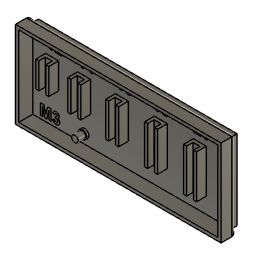
M3 Reference Caliper From 12 v2 (Autodesk Fusion 360 design; units mm, degrees)
Autodesk Fusion 360 part; units mm, degrees
note: some values were not read from the file. Chosen so that the rebuilt part matches the saved one: which bodies a step acts on; which pieces of a blend or face edit are solid.
sketch "Schizzo1" plane through (0, 0, 0) normal (0, 1, 0) x (1, 0, 0)
  line L0 (-43.0702, -47.1256) -> (51.9298, -47.1256)
  line L1 (51.9298, -47.1256) -> (51.9298, -7.1256)
  line L2 (51.9298, -7.1256) -> (-43.0702, -7.1256)
  line L3 (-43.0702, -7.1256) -> (-43.0702, -47.1256)
  line L4 (-34.9398, -37.9923) -> (-30.6504, -37.9923) construction
  line L5 (-30.6504, -37.9923) -> (-30.6504, -43.6096) construction
  line L6 (-30.6504, -43.6096) -> (-34.9398, -43.6096) construction
  line L7 (-34.9398, -43.6096) -> (-34.9398, -37.9923) construction
  line L8 (-20.4362, -37.9923) -> (-16.447, -37.9923) construction
  line L9 (-16.447, -37.9923) -> (-16.447, -43.6096) construction
  line L10 (-16.447, -43.6096) -> (-20.4362, -43.6096) construction
  line L11 (-20.4362, -43.6096) -> (-20.4362, -37.9923) construction
  line L12 (-2.7087, -37.9923) -> (2.1333, -37.9923) construction
  line L13 (2.1333, -37.9923) -> (2.1333, -43.6096) construction
  line L14 (2.1333, -43.6096) -> (-2.7087, -43.6096) construction
  line L15 (-2.7087, -43.6096) -> (-2.7087, -37.9923) construction
  line L16 (14.1885, -37.9923) -> (20.8281, -37.9923) construction
  line L17 (20.8281, -37.9923) -> (20.8281, -43.6096) construction
  line L18 (20.8281, -43.6096) -> (14.1885, -43.6096) construction
  line L19 (14.1885, -43.6096) -> (14.1885, -37.9923) construction
  line L20 (32.7115, -37.9923) -> (40.1532, -37.9923) construction
  line L21 (40.1532, -37.9923) -> (40.1532, -43.6096) construction
  line L22 (40.1532, -43.6096) -> (32.7115, -43.6096) construction
  line L23 (32.7115, -43.6096) -> (32.7115, -37.9923) construction
  line L24 (-35.6629, -35.9305) -> (-29.6629, -35.9305)
  line L25 (-29.6629, -35.9305) -> (-29.6629, -23.9305)
  line L26 (-29.6629, -23.9305) -> (-35.6629, -23.9305)
  line L27 (-35.6629, -23.9305) -> (-35.6629, -35.9305)
  line L28 (-32.6629, -35.9305) -> (-32.6629, -23.9305) construction
  line L29 (-31.0629, -23.9305) -> (-34.2629, -23.9305)
  line L30 (-34.2629, -23.9305) -> (-34.2629, -35.9305)
  line L31 (-34.2629, -35.9305) -> (-31.0629, -35.9305)
  line L32 (-31.0629, -35.9305) -> (-31.0629, -23.9305)
  line L33 (-31.0629, -23.9305) -> (-34.2629, -35.9305) construction
  line L34 (-34.2629, -23.9305) -> (-31.0629, -35.9305) construction
  line L35 (-14.8624, -21.9305) -> (-20.8624, -21.9305)
  line L36 (-19.4624, -21.9305) -> (-16.2624, -35.9305) construction
  line L37 (-16.2624, -21.9305) -> (-19.4624, -21.9305)
  line L38 (-16.2624, -35.9305) -> (-16.2624, -21.9305)
  line L39 (-19.4624, -21.9305) -> (-19.4624, -35.9305)
  line L40 (-16.2624, -21.9305) -> (-19.4624, -35.9305) construction
  line L41 (-17.8624, -35.9305) -> (-17.8624, -21.9305) construction
  line L42 (-20.8624, -35.9305) -> (-14.8624, -35.9305)
  line L43 (-20.8624, -21.9305) -> (-20.8624, -35.9305)
  line L44 (-14.8624, -35.9305) -> (-14.8624, -21.9305)
  line L45 (-19.4624, -35.9305) -> (-16.2624, -35.9305)
  line L46 (1.2, -35.9305) -> (1.2, -19.9305)
  line L47 (-3.4, -19.9305) -> (-3.4, -35.9305)
  line L48 (2.6, -35.9305) -> (2.6, -19.9305)
  line L49 (-3.4, -35.9305) -> (2.6, -35.9305)
  line L50 (1.2, -19.9305) -> (-2, -35.9305) construction
  line L51 (1.2, -19.9305) -> (-2, -19.9305)
  line L52 (-2, -19.9305) -> (-2, -35.9305)
  line L53 (-2, -19.9305) -> (1.2, -35.9305) construction
  line L54 (2.6, -19.9305) -> (-3.4, -19.9305)
  line L55 (-0.4, -35.9305) -> (-0.4, -19.9305) construction
  line L56 (-2, -35.9305) -> (1.2, -35.9305)
  line L57 (16.0001, -35.9305) -> (19.2001, -35.9305)
  line L58 (16.0001, -17.9305) -> (16.0001, -35.9305)
  line L59 (14.6001, -35.9305) -> (20.6001, -35.9305)
  line L60 (19.2001, -35.9305) -> (19.2001, -17.9305)
  line L61 (19.2001, -17.9305) -> (16.0001, -35.9305) construction
  line L62 (20.6001, -17.9305) -> (14.6001, -17.9305)
  line L63 (17.6001, -35.9305) -> (17.6001, -17.9305) construction
  line L64 (14.6001, -17.9305) -> (14.6001, -35.9305)
  line L65 (19.2001, -17.9305) -> (16.0001, -17.9305)
  line L66 (16.0001, -17.9305) -> (19.2001, -35.9305) construction
  line L67 (20.6001, -35.9305) -> (20.6001, -17.9305)
  line L68 (-43.0702, -35.9305) -> (51.9298, -35.9305) construction
  line L69 (32.6049, -35.9305) -> (38.6049, -35.9305)
  line L70 (37.2049, -15.9305) -> (34.0049, -35.9305) construction
  line L71 (38.6049, -35.9305) -> (38.6049, -15.9305)
  line L72 (32.6049, -15.9305) -> (32.6049, -35.9305)
  line L73 (37.2049, -35.9305) -> (37.2049, -15.9305)
  line L74 (37.2049, -15.9305) -> (34.0049, -15.9305)
  line L75 (35.6049, -35.9305) -> (35.6049, -15.9305) construction
  line L76 (34.0049, -15.9305) -> (34.0049, -35.9305)
  line L77 (34.0049, -35.9305) -> (37.2049, -35.9305)
  line L78 (34.0049, -15.9305) -> (37.2049, -35.9305) construction
  line L79 (38.6049, -15.9305) -> (32.6049, -15.9305)
  line L80 (-43.0702, -43.6096) -> (51.9298, -43.6096) construction
  line L81 (50.4298, -45.6256) -> (50.4298, -8.6256)
  line L82 (50.4298, -8.6256) -> (-41.5702, -8.6256)
  line L83 (-41.5702, -8.6256) -> (-41.5702, -45.6256)
  line L84 (-41.5702, -45.6256) -> (50.4298, -45.6256)
  line L85 (-38, -10) -> (-25, -10) construction
  line L86 (-25, -10) -> (-25, -15) construction
  line L87 (-25, -15) -> (-38, -15) construction
  line L88 (-38, -15) -> (-38, -10) construction
  line L89 (-43.0702, -37.9923) -> (50.4298, -37.9923) construction
  circle A0 centre (-17.6072, -12.9667) radius 1.5
  circle A1 centre (-17.6072, -12.9667) radius 2
  point P0 (-32.6629, -29.9305)
  point P1 (-17.8624, -28.9305)
  point P2 (-0.4, -27.9305)
  point P3 (17.6001, -26.9305)
  point P4 (35.6049, -25.9305)
  dimension "d1" = 40
  dimension "d2" = 5
  dimension "d3" = 5
  dimension "d4" = 5
  dimension "d5" = 5
  dimension "d6" = 5
  dimension "d7" = 6
  dimension "d8" = 12
  dimension "d9" = 3.2
  dimension "d21" = 6
  dimension "d22" = 14
  dimension "d23" = 3.2
  dimension "d24" = 6
  dimension "d25" = 16
  dimension "d26" = 3.2
  dimension "d27" = 6
  dimension "d28" = 18
  dimension "d29" = 3.2
  dimension "d30" = 6
  dimension "d31" = 20
  dimension "d32" = 3.2
  dimension "d33" = 95
  dimension "d34" = -1.5
  dimension "d37" = 5
  dimension "d40" = 3
  dimension "d41" = 4
  text T0 "12" font "Arial" height 5 bold align left top in box 4.2894 x 5.6173 at (-34.9398, -37.9923) x (1, 0) y (0, -1) spacing 1
  text T1 "14" font "Arial" height 5 bold align left top in box 3.9891 x 5.6173 at (-20.4362, -37.9923) x (1, 0) y (0, -1) spacing 1
  text T2 "16" font "Arial" height 5 bold align left top in box 4.842 x 5.6173 at (-2.7087, -37.9923) x (1, 0) y (0, -1) spacing 1
  text T3 "18" font "Arial" height 5 bold align left top in box 6.6397 x 5.6173 at (14.1885, -37.9923) x (1, 0) y (0, -1) spacing 1
  text T4 "20" font "Arial" height 5 bold align left top in box 7.4417 x 5.6173 at (32.7115, -37.9923) x (1, 0) y (0, -1) spacing 1
  text T5 "M3" font "Arial" height 5 bold align left top in box 13 x 5 at (-38, -10) x (1, 0) y (0, -1) spacing 1
  constraint horizontal L0
  constraint vertical L1
  constraint horizontal L2
  constraint vertical L3
  constraint horizontal L24
  constraint vertical L25
  constraint horizontal L26
  constraint vertical L27
  constraint midpoint L24 L28.start
  constraint midpoint L26 L28.end
  constraint horizontal L29
  constraint perpendicular L29 L30
  constraint parallel L29 L31
  constraint parallel L30 L32
  constraint coincident L33 P0
  constraint coincident L34 P0
  constraint coincident L26 L29.start
  constraint midpoint L28 P0
  constraint horizontal L42
  constraint vertical L44
  constraint horizontal L35
  constraint vertical L43
  constraint midpoint L41.start L42
  constraint midpoint L41.end L35
  constraint horizontal L37
  constraint perpendicular L37 L39
  constraint parallel L37 L45
  constraint parallel L38 L39
  constraint coincident P1 L40
  constraint coincident P1 L36
  constraint coincident L37.start L35
  constraint midpoint P1 L41
  constraint horizontal L49
  constraint vertical L48
  constraint horizontal L54
  constraint vertical L47
  constraint midpoint L55.start L49
  constraint midpoint L55.end L54
  constraint horizontal L51
  constraint perpendicular L51 L52
  constraint parallel L51 L56
  constraint parallel L46 L52
  constraint coincident P2 L50
  constraint coincident P2 L53
  constraint coincident L46.end L54
  constraint midpoint P2 L55
  constraint horizontal L59
  constraint vertical L67
  constraint horizontal L62
  constraint vertical L64
  constraint midpoint L63.start L59
  constraint midpoint L63.end L62
  constraint horizontal L65
  constraint perpendicular L58 L65
  constraint parallel L57 L65
  constraint parallel L58 L60
  constraint coincident P3 L61
  constraint coincident P3 L66
  constraint coincident L60.end L62
  constraint midpoint P3 L63
  constraint coincident L3 L68.start
  constraint coincident L1 L68.end
  constraint perpendicular L1 L68
  constraint collinear L31 L68
  constraint collinear L49 L68
  constraint collinear L59 L68
  constraint horizontal L69
  constraint vertical L71
  constraint horizontal L79
  constraint vertical L72
  constraint midpoint L75.start L69
  constraint midpoint L75.end L79
  constraint horizontal L74
  constraint perpendicular L74 L76
  constraint parallel L74 L77
  constraint parallel L73 L76
  constraint coincident P4 L70
  constraint coincident P4 L78
  constraint coincident L70.start L79
  constraint midpoint P4 L75
  constraint coincident L3 L80.start
  constraint coincident L1 L80.end
  constraint perpendicular L1 L80
  constraint collinear L42 L68
  constraint collinear L68 L69
  constraint collinear L6 L80
  constraint collinear L10 L80
  constraint collinear L14 L80
  constraint collinear L18 L80
  constraint collinear L22 L80
  constraint coincident L3 L89.start
  constraint coincident L81 L89.end
  constraint perpendicular L81 L89
  constraint collinear L4 L89
  constraint collinear L8 L89
  constraint collinear L12 L89
  constraint collinear L16 L89
  constraint collinear L20 L89
  constraint concentric A0 A1
  measures "d1" distance of L0 L2
  measures "d7" distance of L24.start L24.end
  measures "d8" distance of L24.start L26.end
  measures "d9" distance of L30 L32
  measures "d21" distance of L42.start L42.end
  measures "d22" distance of L42.start L35.end
  measures "d23" distance of L38 L39
  measures "d24" distance of L47.end L48.start
  measures "d25" distance of L47.start L47.end
  measures "d26" distance of L46 L52
  measures "d27" distance of L59.end L59.start
  measures "d28" distance of L62.end L59.start
  measures "d29" distance of L58 L60
  measures "d30" distance of L69.start L69.end
  measures "d31" distance of L69.start L72.start
  measures "d32" distance of L73 L76
  measures "d33" distance of L1 L3
  measures "d40" diameter of A0
  measures "d41" diameter of A1
extrude "Estrusione1" add sketch "Schizzo1" along normal blind 0.4 text T0 T1 T2 T3 T4 T5 makes body 1 at (-33.0628, 0, 41.4871) makes body 2 at (39.618, 0, 40.7205) makes body 3 at (1.6347, 0, 41.0707) makes body 4 at (-14.3095, 0, 42.0851) makes body 5 at (19.8593, 0, 41.2901) makes body 6 at (34.3168, 0, 38.9063) makes body 7 at (-30.4309, 0, 12.6932) makes body 8 at (-37.6874, 0, 12.9786) makes body 9 at (-29.8283, 0, 38.9063) makes body 10 at (-18.5592, 0, 41.4871) makes body 11 at (-0.8317, 0, 41.4871) makes body 12 at (16.0655, 0, 41.4871)
extrude "Estrusione2" add sketch "Schizzo1" along normal blind 0.5 separate body contours L0 L1 L2 L3 | L24 L26 L27 L30 | L24 L26 L29 L30 L31 L32 | L24 L25 L26 L32 | L35 L38 L42 L44 | L35 L37 L38 L39 L42 L45 | L35 L39 L42 L43 | L46 L49 L51 L52 L54 L56 | L46 L48 L49 L54 | L47 L49 L52 L54 | L57 L58 L59 L60 L62 L65 | L58 L59 L62 L64 | L59 L60 L62 L67 | L69 L72 L76 L79 | L69 L73 L74 L76 L77 L79 | L69 L71 L73 L79 | L81 L82 L83 L84 | A0 | A1 makes body 13
extrude "Estrusione7" cut sketch "Schizzo1" along normal blind 0.4 text T0 T1 T2 T3 T5 T4 bodies 13
extrude "Estrusione6" add sketch "Schizzo1" against normal blind 6.5 contours L0 L1 L2 L3 bodies 13
extrude "Estrusione4" add sketch "Schizzo1" against normal blind 4.5 contours L24 L26 L27 L30 | L24 L26 L29 L30 L31 L32 | L24 L25 L26 L32 | L35 L38 L42 L44 | L35 L37 L38 L39 L42 L45 | L35 L39 L42 L43 | L46 L49 L51 L52 L54 L56 | L46 L48 L49 L54 | L47 L49 L52 L54 | L57 L58 L59 L60 L62 L65 | L58 L59 L62 L64 | L59 L60 L62 L67 | L69 L72 L76 L79 | L69 L73 L74 L76 L77 L79 | L69 L71 L73 L79 | A0 bodies 13
extrude "Estrusione8" add sketch "Schizzo1" against normal blind 1 contours A1 bodies 13
extrude "Estrusione5" cut sketch "Schizzo1" along normal blind 3 from surface at -4.5 contours L24 L26 L29 L30 L31 L32 | L35 L37 L38 L39 L42 L45 | L46 L49 L51 L52 L54 L56 | L57 L58 L59 L60 L62 L65 | L69 L73 L74 L76 L77 L79 bodies 13
sketch "Schizzo2" plane through (0, 0.5, 0) normal (0, 1, 0) x (-1, 0, 0)
  line L0 (43.0702, 7.1256) -> (43.0702, 47.1256)
  line L1 (43.0702, 47.1256) -> (-51.9298, 47.1256)
  line L2 (-51.9298, 47.1256) -> (-51.9298, 7.1256)
  line L3 (-51.9298, 7.1256) -> (43.0702, 7.1256)
  line L4 (-51.9298, 47.1256) -> (43.0702, 47.1256) construction
  line L5 (43.0702, 47.1256) -> (43.0702, 7.1256) construction
  line L6 (43.0702, 7.1256) -> (-51.9298, 7.1256) construction
  line L7 (-51.9298, 7.1256) -> (-51.9298, 47.1256) construction
  line L8 (43.0702, 47.1256) -> (-51.9298, 47.1256) construction
  line L9 (-51.9298, 47.1256) -> (-51.9298, 7.1256) construction
  line L10 (-51.9298, 7.1256) -> (43.0702, 7.1256) construction
  line L11 (43.0702, 7.1256) -> (43.0702, 47.1256) construction
  line L12 (-51.9298, 27.1256) -> (-50, 27.1256) construction
  line L13 (-50, 27.1256) -> (43.0702, 27.1256) construction
  line L14 (-4.4298, 47.1256) -> (-4.4298, 7.1256) construction
  line L15 (41.4702, 8.7256) -> (-50.3298, 8.7256)
  line L16 (-50.3298, 8.7256) -> (-50.3298, 45.5256)
  line L17 (-50.3298, 45.5256) -> (41.4702, 45.5256)
  line L18 (41.4702, 45.5256) -> (41.4702, 8.7256)
  line L19 (41.4702, 8.7256) -> (-50.3298, 45.5256) construction
  line L20 (-50.3298, 8.7256) -> (41.4702, 45.5256) construction
  point P0 (-4.4298, 27.1256)
  dimension "d44" = 1.6
  dimension "d45" = 1.6
  constraint horizontal L4
  constraint vertical L5
  constraint horizontal L6
  constraint vertical L7
  constraint collinear L4 L8
  constraint collinear L7 L9
  constraint collinear L6 L10
  constraint collinear L5 L11
  constraint midpoint L9 L12.start
  constraint perpendicular L9 L12
  constraint midpoint L11 L13.end
  constraint perpendicular L11 L13
  constraint midpoint L4 L14.start
  constraint midpoint L6 L14.end
  constraint horizontal L15
  constraint perpendicular L15 L16
  constraint parallel L15 L17
  constraint parallel L16 L18
  constraint coincident L19 P0
  constraint coincident L20 P0
  constraint midpoint L14 P0
  measures "d44" distance of L7 L16
  measures "d45" distance of L4 L17
extrude "Estrusione9" add sketch "Schizzo2" along normal blind 2 contours L15 L16 L17 L18 bodies 13
fillet "Raccordo1" radius 2 4 edges at (4.4298, 0.5, 7.1256) (51.9298, 0.5, 27.1256) (-43.0702, 0.5, 27.1256) (4.4298, 0.5, 47.1256) on bodies 13
equation "d21 = d7"
equation "d23 = d9"
equation "d24 = d7"
equation "d26 = d9"
equation "d27 = d7"
equation "d29 = d9"
equation "d30 = d7"
equation "d32 = d9"
equation "d45 = d44"
